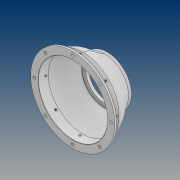
# Autodesk Inventor part: kelyfos_2
Saved by Autodesk Inventor 2021 (Build 250183000, 183)
## iProperties
Created: 2020-12-27
Part Number: kelyfos_2
Material: Generic
Document SubType Name: Modeling
Designer: Angelos
Density: 1 g/cm^3
Appearance: Default
Mass: 17147.3 g
Surface Area: 20216.9 cm^2
Volume: 17147.3 cm^3
Author: Angelos
Autodesk Inventor part; units mm, degrees
ref_plane "YZ Plane" through (0, 0, 0) normal (1, 0, 0) x (0, 1, 0)
ref_plane "XZ Plane" through (0, 0, 0) normal (0, 1, 0) x (-1, 0, 0)
sketch "Sketch1" plane through (0, 0, 0) normal (0, 0, 1) x (1, 0, 0)
  circle A0 centre (0, 0) radius 465
  circle A1 centre (0, 0) radius 381
  circle A2 centre (0, 425) radius 15
  dimension "d0" = 930
  dimension "d1" = 762
  dimension "d2" = 30
  dimension "d3" = 0
  dimension "d4" = 425
  constraints: 3 centre point, 2 coincident
  measures "d0" diameter of A0
  measures "d1" diameter of A1
  measures "d2" diameter of A2
  measures "d3" horizontal distance of point (0, 0) A2.centre
  measures "d4" distance of point (0, 0) A2.centre
extrude "Extrusion1" add sketch "Sketch1" along normal blind 20 contours A0 | A2
extrude "Extrusion2" cut sketch "Sketch1" along normal blind 20 contours A2
pattern_circular "Circular Pattern1" count 8 over 360 about axis through (0, 0, -10) along (0, 0, 1) of "Extrusion2"
sketch "Sketch2" plane through (0, 0, 0) normal (0, 0, -1) x (-1, 0, 0)
  circle A0 centre (0, 0) radius 381
  circle A1 centre (0, 0) radius 401
  dimension "d12" = 762
  dimension "d13" = 802
  constraints: 2 centre point, 2 coincident
  measures "d12" diameter of A0
  measures "d13" diameter of A1
extrude "Extrusion3" add sketch "Sketch2" along normal blind 90
sketch "Sketch3" plane through (0, 0, 0) normal (1, 0, 0) x (0, 1, 0)
  line L0 (-401, -90) -> (401, -90) projected
  line L1 (401, -90) -> (531, -90) construction
  line L2 (381, -90) -> (-381, -90) projected
  line L3 (0, -491.3111) -> (0, 105.2185) projected
  line L4 (0, 0) -> (0, -215)
  line L5 (381, 20) -> (381, -90) projected
  line L6 (381, -90) -> (401, -90)
  line L7 (401, 0) -> (401, -60) projected
  line L8 (0, 0) -> (0, -338.278)
  line L9 (0, -360.278) -> (0, -338.278)
  line L10 (246.068, -328.278) -> (267.9668, -328.278)
  line L11 (-381, 20) -> (381, 20) projected
  line L12 (381, 20) -> (381, -360.278)
  line L13 (381, -360.278) -> (0, -360.278)
  line L14 (267.9668, -328.278) -> (0, -328.278)
  spline S0 degree 3 poles (401, -90) (382.934, -208.4386) (299.528, -242.0386) (267.9668, -328.278) knots 0 0 0 0 1 1 1 1
  line L15 (381, -90) -> (401, -90)
  spline S1 degree 3 poles (381, -90) (362.934, -208.4385) (279.528, -242.0386) (247.9668, -328.278) knots 0 0 0 0 1 1 1 1
  point P0 (360.4578, -192.9789)
  point P1 (309.6369, -258.0596)
  point P2 (381, -156.966)
  point P3 (340.4579, -192.9789)
  point P4 (289.6369, -258.0596)
  point P5 (247.9668, -328.278)
  constraints: 20 end point, 4 perpendicular, 2 collinear, 2 point on line, 1 horizontal, 1 vertical, 9 other
sketch "Sketch8" plane through (0, 0, 0) normal (1, 0, 0) x (0, 1, 0)
  line L0 (0, -432.3336) -> (0, 72.0556) projected
  line L1 (0, 0) -> (0, -360.278)
  line L2 (203.2661, -360.278) -> (266.068, -360.278)
  line L3 (203.2661, -338.278) -> (203.2661, -360.278)
  line L4 (203.2661, -360.278) -> (203.2661, -338.278)
  line L5 (203.2661, -338.278) -> (203.2661, -328.278)
  line L6 (203.2661, -328.278) -> (266.068, -328.278)
  line L7 (266.068, -360.278) -> (267.967, -360.278)
  line L8 (267.967, -360.278) -> (267.967, -328.278)
  line L9 (267.967, -328.278) -> (266.068, -328.278)
  line L10 (465, 20) -> (-465, 20) projected
  line L11 (0, 20) -> (0, -360.278)
  constraints: 20 end point, 4 perpendicular, 2 collinear, 1 horizontal, 1 midpoint, 1 point on line, 1 vertical
revolve "Revolution6" add sketch "Sketch8" angle 360 about axis through (0, 0, -10) along (0, 0, 1)
ref_plane "Work Plane2" through (0, 0, -360.278) normal (0, 0, -1) x (-1, 0, 0)
revolve "Revolution7" add sketch "Sketch3" angle 360 about axis through (0, 0, -10) along (0, 0, 1) contours L0 S0 L12 | L12 S0 L10 S1
sketch "Sketch13" plane through (0, 0, -360.278) normal (0, 0, -1) x (-1, 0, 0)
  circle A0 centre (0, 0) radius 232.5
  circle A1 centre (0, 232.5) radius 12.5
  dimension "d108" = 465
  dimension "d109" = 25
  constraints: 1 centre point, 1 coincident, 1 vertical alignment, 2 other
  measures "d109" diameter of A1
extrude "Extrusion7" cut sketch "Sketch13" against normal blind 15 contours A1 A0 | A0 A1 picked at (0.4937, 228.3378) picked at (0.4509, 236.6173)
pattern_circular "Circular Pattern5" count 6 over 360 about axis through (0, 0, -10) along (0, 0, 1) of "Extrusion7"
sketch "Sketch14" plane through (0, 0, 0) normal (1, 0, 0) x (0, 1, 0)
  line L0 (245, -345.278) -> (220, -345.278) projected
  line L1 (220, -345.278) -> (232.5, -345.278)
  line L2 (232.5, -345.278) -> (232.5, -337.278)
  line L3 (232.5, -337.278) -> (220, -345.278)
  point P0 (0, 0)
  constraints: 6 end point, 1 collinear, 1 perpendicular
revolve "Revolution8" cut sketch "Sketch14" angle 360 about axis through (0, 232.5, -345.278) along (0, 0, 1)
pattern_circular "Circular Pattern6" count 6 over 360 about axis through (0, 0, -10) along (0, 0, 1) of "Revolution8"
sketch "Sketch15" plane through (0, 0, 0) normal (0, 1, 0) x (-1, 0, 0)
  circle A0 centre (0, -60) radius 10.5
  point P0 (0, 0)
  dimension "d119" = 21
  dimension "d120" = 0
  dimension "d121" = 60
  constraints: 1 centre point
  measures "d119" diameter of A0
  measures "d120" horizontal distance of point (0, 0) A0.centre
  measures "d121" distance of point (0, 0) A0.centre
extrude "Extrusion8" cut sketch "Sketch15" along normal through all
pattern_circular "Circular Pattern7" count 8 over 360 about axis through (0, 0, -10) along (0, 0, 1) of "Extrusion8"
thread "Thread13" size "M22x3" class "6H" standard "ANSI Metric M Profile" full length
thread "Thread14" size "M22x3" class "6H" standard "ANSI Metric M Profile" full length
thread "Thread15" size "M22x3" class "6H" standard "ANSI Metric M Profile" full length
thread "Thread16" size "M22x3" class "6H" standard "ANSI Metric M Profile" full length
thread "Thread17" size "M25x2" class "6H" standard "ANSI Metric M Profile" full length
thread "Thread18" size "M25x2" class "6H" standard "ANSI Metric M Profile" full length
thread "Thread19" size "M25x2" class "6H" standard "ANSI Metric M Profile" full length
thread "Thread20" size "M25x2" class "6H" standard "ANSI Metric M Profile" full length
thread "Thread21" size "M25x2" class "6H" standard "ANSI Metric M Profile" full length
thread "Thread22" size "M25x2" class "6H" standard "ANSI Metric M Profile" full length
fillet "Fillet4" radius 3 1 edges at (0, -247.9668, -328.278)
fillet "Fillet5" radius 3 1 edges at (-381, 0, 20)
fillet "Fillet6" radius 3 1 edges at (401, 0, 0)
body "Solid1"
